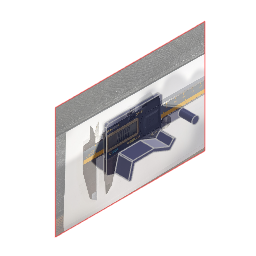
caliper stand (Autodesk Fusion 360 design; units mm, degrees)
Autodesk Fusion 360 part; units mm, degrees
sketch "Sketch1" plane through (0, 0, 0) normal (1, 0, 0) x (0, 1, 0)
  line L0 (-5.19, -7.01) -> (-3.78, -7)
  line L1 (-13, -16.1) -> (11.5, -15.8)
  line L2 (27.8164, -22.4078) -> (11.5, -15.8)
  line L3 (27.8164, -22.4078) -> (31.6352, -18.1647)
  line L4 (-13, -16.1) -> (-17.5, -34)
  line L5 (-12.7967, -17.3419) -> (-16.7713, -33.1521)
  line L6 (-11.8391, -16.5858) -> (11.2044, -16.3037)
  line L7 (27.9536, -23.0028) -> (11.592, -16.3767)
  line L8 (27.9536, -23.0028) -> (32.7851, -17.6344)
  line L9 (-10.0593, -20.8087) -> (-13.3769, -34.0054)
  line L10 (-9.1017, -20.0526) -> (10.5432, -19.812)
  line L11 (28.2641, -26.9047) -> (10.9308, -19.8851)
  line L12 (29.3828, -26.6468) -> (35.3866, -19.9758)
  arc A0 (-11.8391, -16.5858) -> (-12.7967, -17.3419) centre (-11.8268, -17.5857) ccw
  arc A1 (11.592, -16.3767) -> (11.2044, -16.3037) centre (11.2166, -17.3036) ccw
  arc A2 (28.2641, -26.9047) -> (29.3828, -26.6468) centre (28.6395, -25.9778) ccw
  arc A3 (-9.1017, -20.0526) -> (-10.0593, -20.8087) centre (-9.0895, -21.0525) ccw
  arc A4 (10.9308, -19.8851) -> (10.5432, -19.812) centre (10.5555, -20.8119) ccw
  line L13 (-16.0453, -34.3657) -> (-14.5905, -34.7314)
  line L14 (35.3123, -18.5635) -> (34.1974, -17.5601)
  arc A5 (34.1974, -17.5601) -> (32.7851, -17.6344) centre (33.5284, -18.3034) ccw
  arc A6 (35.3866, -19.9758) -> (35.3123, -18.5635) centre (34.6433, -19.3068) ccw
  arc A7 (-16.7713, -33.1521) -> (-16.0453, -34.3657) centre (-15.8015, -33.3959) ccw
  arc A8 (-14.5905, -34.7314) -> (-13.3769, -34.0054) centre (-14.3467, -33.7616) ccw
  circle A9 centre (57, -12.25) radius 4
  dimension "d4" = 1
  dimension "d5" = 1
  dimension "d34" = 8
  dimension "d41" = 12.25
  dimension "d42" = 57
  constraint parallel L4 L5
  constraint parallel L1 L6
  constraint parallel L2 L7
  constraint parallel L3 L8
  constraint tangent L6 A0
  constraint tangent L5 A0
  constraint tangent L6 A1
  constraint tangent L7 A1
  constraint equal A0 A1
  constraint parallel L4 L9
  constraint parallel L1 L10
  constraint parallel L2 L11
  constraint parallel L3 L12
  constraint tangent L12 A2
  constraint tangent L11 A2
  constraint equal A0 A2
  constraint tangent L10 A3
  constraint tangent L9 A3
  constraint equal A0 A3
  constraint tangent L10 A4
  constraint tangent L11 A4
  constraint equal A0 A4
  constraint perpendicular L9 L13
  constraint perpendicular L8 L14
  constraint tangent L8 A5
  constraint tangent L14 A5
  constraint tangent L12 A6
  constraint tangent L14 A6
  constraint equal A5 A6
  constraint tangent L13 A7
  constraint tangent L5 A7
  constraint equal A5 A7
  constraint tangent L13 A8
  constraint tangent L9 A8
  constraint equal A5 A8
  measures "d4" radius of A0
  measures "d5" radius of A5
  measures "d34" diameter of A9
  measures "d41" vertical distance of origin A9.centre
  measures "d42" horizontal distance of origin A9.centre
extrude "Extrude1" add sketch "Sketch1" along normal blind 15 makes body 1 at (5, -4.1579, -16.4918) makes body 2 at (10, 60.9801, -12.6483)
sketch "Sketch3" plane through (0, 0, 0) normal (1, 0, 0) x (0, 1, 0)
  line L0 (28.2641, -26.9047) -> (10.9308, -19.8851)
  arc A0 (28.2641, -26.9047) -> (29.3828, -26.6468) centre (28.6395, -25.9778) ccw
  line L1 (29.3828, -26.6468) -> (35.3866, -19.9758)
  line L2 (-9.1017, -20.0526) -> (10.5432, -19.812)
  line L3 (-10.0593, -20.8087) -> (-13.3769, -34.0054)
  arc A1 (-9.1017, -20.0526) -> (-10.0593, -20.8087) centre (-9.0895, -21.0525) ccw
  arc A2 (-14.5905, -34.7314) -> (-13.3769, -34.0054) centre (-14.3467, -33.7616) ccw
  line L4 (-16.0453, -34.3657) -> (-14.5905, -34.7314)
  arc A3 (-16.7713, -33.1521) -> (-16.0453, -34.3657) centre (-15.8015, -33.3959) ccw
  line L5 (-12.7967, -17.3419) -> (-16.7713, -33.1521)
  line L6 (35.3866, 7.7018) -> (35.3866, 14)
  line L7 (32.3866, 17) -> (-23, 17)
  line L8 (-26, 14) -> (-26, -29.524)
  line L9 (-23.7314, -32.4334) -> (-16.0453, -34.3657)
  arc A4 (-26, -29.524) -> (-23.7314, -32.4334) centre (-23, -29.524) ccw
  arc A5 (-23, 17) -> (-26, 14) centre (-23, 14) ccw
  arc A6 (35.3866, 14) -> (32.3866, 17) centre (32.3866, 14) ccw
  line L10 (35.3866, -19.9758) -> (29.3828, -26.6468)
  line L11 (28.2641, -26.9047) -> (10.9308, -19.8851)
  line L12 (-9.1017, -20.0526) -> (10.5432, -19.812)
  line L13 (-10.0593, -20.8087) -> (-13.3769, -34.0054)
  line L14 (-14.5905, -34.7314) -> (-16.0453, -34.3657)
  arc A7 (28.2641, -26.9047) -> (29.3828, -26.6468) centre (28.6395, -25.9778) ccw
  arc A8 (10.9308, -19.8851) -> (10.5432, -19.812) centre (10.5555, -20.8119) ccw
  arc A9 (10.9308, -19.8851) -> (10.5432, -19.812) centre (10.5555, -20.8119) ccw
  arc A10 (-9.1017, -20.0526) -> (-10.0593, -20.8087) centre (-9.0895, -21.0525) ccw
  arc A11 (-14.5905, -34.7314) -> (-13.3769, -34.0054) centre (-14.3467, -33.7616) ccw
  line L15 (-10, 17) -> (-10, 14)
  line L16 (-10, 14) -> (-26, 14)
  circle A12 centre (57, -12.25) radius 4
  line L17 (57, -16.25) -> (36.3866, -16.25)
  line L18 (59.3943, -9.0457) -> (37.8866, 3.3717)
  arc A13 (35.3866, 7.7018) -> (37.8866, 3.3717) centre (40.3866, 7.7018) ccw
  line L19 (35.3866, -19.9758) -> (35.3866, -17.25)
  arc A14 (36.3866, -16.25) -> (35.3866, -17.25) centre (36.3866, -17.25) ccw
  arc A15 (57, -16.25) -> (59.3943, -9.0457) centre (57, -12.25) ccw
  point P0 (-16.0453, -34.3657)
  dimension "d8" = 3
  dimension "d35" = 30
  dimension "d36" = 5
  dimension "d37" = 1
  constraint vertical L6
  constraint perpendicular L6 L7
  constraint perpendicular L7 L8
  constraint coincident P0 L4.start
  constraint collinear L4 L9
  constraint tangent L9 A4
  constraint tangent L8 A4
  constraint tangent L8 A5
  constraint tangent L7 A5
  constraint equal A4 A5
  constraint tangent L7 A6
  constraint tangent L6 A6
  constraint equal A4 A6
  constraint coincident L1.end L10.start
  constraint coincident A0.end L1.start
  constraint coincident L0.start A0.start
  constraint coincident L0.end L11.end
  constraint coincident L2.start A1.start
  constraint coincident L2.end L12.end
  constraint coincident L3.start A1.end
  constraint coincident L3.end A2.end
  constraint coincident A2.start L4.end
  constraint coincident A0.centre A7.centre
  constraint coincident A2.centre A11.centre
  constraint coincident L7 L15.start
  constraint perpendicular L7 L15
  constraint coincident A12 L17.start
  constraint tangent A12 L17
  constraint horizontal L17
  constraint coincident A12 L18.start
  constraint tangent L18 A13
  constraint tangent L6 A13
  constraint perpendicular L17 L19
  constraint tangent L19 A14
  constraint tangent L17 A14
  constraint coincident A12.centre A15.centre
  measures "d8" radius of A4
  measures "d35" angle of L17 L18
  measures "d36" radius of A13
  measures "d37" radius of A14
extrude "Extrude2" add sketch "Sketch3" against normal blind 3 contours L0 A0 L1 L2 L3 A1 A2 L4 L6 L7 L8 L9 A4 A6 L10 L11 L12 L13 L14 A7 A8 A9 A10 A11 L15 L16 A12 L17 L18 A13 L19 A14 | A12 L18 A15 | L7 A5 L15 L16 bodies 1 2
ref_plane "WorkPlane1" through (0, 12.125, 0) normal (0.34202, 0, 0.939693) x (0, 1, 0)
sketch "Sketch4" plane through (0, 12.125, 0) normal (0.34202, 0, 0.939693) x (0, 1, 0)
  ellipse E0 centre (-35.125, 4.7883) end of major axis (-38.125, 4.7883) minor radius 1.0261 (-35.125, 5.8143) -> (-38.125, 4.7883) ccw
  line L0 (-35.125, 5.8143) -> (-35.125, 8.6334)
  ellipse E1 centre (-35.125, 7.6074) end of major axis (-38.125, 7.6074) minor radius 1.0261 (-35.125, 8.6334) -> (-38.125, 7.6074) ccw
  line L1 (-38.125, 7.6074) -> (-38.125, 4.7883)
  line L2 (-35.125, 5.8143) -> (20.2616, 5.8143)
  line L3 (20.2616, 5.8143) -> (20.2616, 8.6334)
  line L4 (20.2616, 8.6334) -> (-35.125, 8.6334)
  ellipse E2 centre (20.2616, 4.7883) end of major axis (23.2616, 4.7883) minor radius 1.0261 (23.2616, 4.7883) -> (20.2616, 5.8143) ccw
  line L5 (23.2616, 4.7883) -> (23.2616, 7.6074)
  ellipse E3 centre (20.2616, 7.6074) end of major axis (23.2616, 7.6074) minor radius 1.0261 (23.2616, 7.6074) -> (20.2616, 8.6334) ccw
  line L6 (20.2616, 8.6334) -> (20.2616, 5.8143)
  ellipse E4 centre (22.5183, -6.6033) end of major axis (21.5183, -6.6033) minor radius 0.342 (23.2616, -6.3745) -> (23.1873, -6.3491) ccw
  line L7 (23.2616, 2.6342) -> (23.2616, 4.7883)
  ellipse E5 centre (20.2616, 4.7883) end of major axis (23.2616, 4.7883) minor radius 1.0261 (23.2616, 4.7883) -> (20.2616, 5.8143) ccw
  line L8 (20.2616, 5.8143) -> (-35.125, 5.8143)
  line L9 (-38.125, 4.7883) -> (-38.125, -10.0978)
  ellipse E6 centre (-35.125, -10.0978) end of major axis (-38.125, -10.0978) minor radius 1.0261 (-38.125, -10.0978) -> (-35.8564, -11.0929) ccw
  line L10 (-35.8564, -11.0929) -> (-28.1703, -11.7538)
  ellipse E7 centre (-27.9265, -11.4221) end of major axis (-28.9265, -11.4221) minor radius 0.342 (-28.8963, -11.3387) -> (-28.1703, -11.7538) ccw
  line L11 (-28.8963, -11.3387) -> (-24.9217, -5.9313)
  ellipse E8 centre (-23.9518, -6.0147) end of major axis (-24.9518, -6.0147) minor radius 0.342 (-23.9641, -5.6727) -> (-24.9217, -5.9313) ccw
  line L12 (-23.9641, -5.6727) -> (-0.9206, -5.5762)
  ellipse E9 centre (-0.9084, -5.9182) end of major axis (-1.9084, -5.9182) minor radius 0.342 (-0.533, -5.6012) -> (-0.9206, -5.5762) ccw
  line L13 (-0.533, -5.6012) -> (15.8286, -7.8674)
  line L14 (15.8286, -7.8674) -> (20.6601, -6.0313)
  ellipse E10 centre (21.4034, -6.2601) end of major axis (20.4034, -6.2601) minor radius 0.342 (22.0724, -6.0059) -> (20.6601, -6.0313) ccw
  line L15 (22.0724, -6.0059) -> (23.1873, -6.3491)
  line L16 (-35.125, 8.6334) -> (20.2616, 8.6334)
  line L17 (20.2616, 8.6334) -> (20.2616, 0.6334)
  line L18 (20.2616, 0.6334) -> (-35.125, 0.6334)
  line L19 (-35.125, 0.6334) -> (-35.125, 8.6334)
  line L20 (23.2616, -6.3745) -> (23.2616, -5.8998)
  ellipse E11 centre (24.2616, -5.8998) end of major axis (23.2616, -5.8998) minor radius 0.342 (24.2616, -5.5578) -> (23.2616, -5.8998) ccw
  line L21 (24.2616, -5.5578) -> (44.875, -5.5578)
  line L22 (46.4528, -2.9326) -> (25.7616, 1.1532)
  ellipse E12 centre (28.2616, 2.6342) end of major axis (23.2616, 2.6342) minor radius 1.7101 (23.2616, 2.6342) -> (25.7616, 1.1532) ccw
  line L23 (-35.125, 8.6334) -> (-35.125, 5.8143)
  ellipse E13 centre (-35.125, 4.7883) end of major axis (-38.125, 4.7883) minor radius 1.0261 (-35.125, 5.8143) -> (-38.125, 4.7883) ccw
  ellipse E14 centre (44.875, -4.1897) end of major axis (40.875, -4.1897) minor radius 1.3681 (46.4528, -2.9326) -> (44.875, -5.5578) ccw
  dimension "d12" = 8
  constraint perpendicular L16 L17
  constraint parallel L16 L18
  constraint parallel L17 L19
  constraint coincident L3.end L4.start
  constraint perpendicular L3 L16
  constraint coincident L0.end L4.end
  measures "d12" distance of L0.end L18.end
ref_plane "WorkPlane2" through (-11.6287, 12.125, -31.9495) normal (0.34202, 0, 0.939693) x (0, 1, 0)
sketch "Sketch5" plane through (-11.6287, 12.125, -31.9495) normal (0.34202, 0, 0.939693) x (0, 1, 0)
  ellipse E0 centre (-35.125, 4.7883) end of major axis (-38.125, 4.7883) minor radius 1.0261 (-35.125, 5.8143) -> (-38.125, 4.7883) ccw
  line L0 (-35.125, 5.8143) -> (-35.125, 8.6334)
  ellipse E1 centre (-35.125, 7.6074) end of major axis (-38.125, 7.6074) minor radius 1.0261 (-35.125, 8.6334) -> (-38.125, 7.6074) ccw
  line L1 (-38.125, 7.6074) -> (-38.125, 4.7883)
  line L2 (-35.125, 5.8143) -> (20.2616, 5.8143)
  line L3 (20.2616, 5.8143) -> (20.2616, 8.6334)
  line L4 (20.2616, 8.6334) -> (-35.125, 8.6334)
  ellipse E2 centre (20.2616, 4.7883) end of major axis (23.2616, 4.7883) minor radius 1.0261 (23.2616, 4.7883) -> (20.2616, 5.8143) ccw
  line L5 (23.2616, 4.7883) -> (23.2616, 7.6074)
  ellipse E3 centre (20.2616, 7.6074) end of major axis (23.2616, 7.6074) minor radius 1.0261 (23.2616, 7.6074) -> (20.2616, 8.6334) ccw
  line L6 (20.2616, 8.6334) -> (20.2616, 5.8143)
  ellipse E4 centre (22.5183, -6.6033) end of major axis (21.5183, -6.6033) minor radius 0.342 (23.2616, -6.3745) -> (23.1873, -6.3491) ccw
  line L7 (23.2616, 2.6342) -> (23.2616, 4.7883)
  ellipse E5 centre (20.2616, 4.7883) end of major axis (23.2616, 4.7883) minor radius 1.0261 (23.2616, 4.7883) -> (20.2616, 5.8143) ccw
  line L8 (20.2616, 5.8143) -> (-35.125, 5.8143)
  line L9 (-38.125, 4.7883) -> (-38.125, -10.0978)
  ellipse E6 centre (-35.125, -10.0978) end of major axis (-38.125, -10.0978) minor radius 1.0261 (-38.125, -10.0978) -> (-35.8564, -11.0929) ccw
  line L10 (-35.8564, -11.0929) -> (-28.1703, -11.7538)
  ellipse E7 centre (-27.9265, -11.4221) end of major axis (-28.9265, -11.4221) minor radius 0.342 (-28.8963, -11.3387) -> (-28.1703, -11.7538) ccw
  line L11 (-28.8963, -11.3387) -> (-24.9217, -5.9313)
  ellipse E8 centre (-23.9518, -6.0147) end of major axis (-24.9518, -6.0147) minor radius 0.342 (-23.9641, -5.6727) -> (-24.9217, -5.9313) ccw
  line L12 (-23.9641, -5.6727) -> (-0.9206, -5.5762)
  ellipse E9 centre (-0.9084, -5.9182) end of major axis (-1.9084, -5.9182) minor radius 0.342 (-0.533, -5.6012) -> (-0.9206, -5.5762) ccw
  line L13 (-0.533, -5.6012) -> (15.8286, -7.8674)
  line L14 (15.8286, -7.8674) -> (20.6601, -6.0313)
  ellipse E10 centre (21.4034, -6.2601) end of major axis (20.4034, -6.2601) minor radius 0.342 (22.0724, -6.0059) -> (20.6601, -6.0313) ccw
  line L15 (22.0724, -6.0059) -> (23.1873, -6.3491)
  line L16 (-35.125, 8.6334) -> (20.2616, 8.6334)
  line L17 (20.2616, 8.6334) -> (20.2616, 0.6334)
  line L18 (20.2616, 0.6334) -> (-35.125, 0.6334)
  line L19 (-35.125, 0.6334) -> (-35.125, 8.6334)
  line L20 (23.2616, -6.3745) -> (23.2616, -5.8998)
  ellipse E11 centre (24.2616, -5.8998) end of major axis (23.2616, -5.8998) minor radius 0.342 (24.2616, -5.5578) -> (23.2616, -5.8998) ccw
  line L21 (24.2616, -5.5578) -> (44.875, -5.5578)
  line L22 (46.4528, -2.9326) -> (25.7616, 1.1532)
  ellipse E12 centre (28.2616, 2.6342) end of major axis (23.2616, 2.6342) minor radius 1.7101 (23.2616, 2.6342) -> (25.7616, 1.1532) ccw
  line L23 (-35.125, 8.6334) -> (-35.125, 5.8143)
  ellipse E13 centre (-35.125, 4.7883) end of major axis (-38.125, 4.7883) minor radius 1.0261 (-35.125, 5.8143) -> (-38.125, 4.7883) ccw
  ellipse E14 centre (44.875, -4.1897) end of major axis (40.875, -4.1897) minor radius 1.3681 (46.4528, -2.9326) -> (44.875, -5.5578) ccw
  dimension "d14" = 8
  constraint perpendicular L16 L17
  constraint parallel L16 L18
  constraint parallel L17 L19
  constraint coincident L3.end L4.start
  constraint tangent E1 L16
  constraint coincident L0.end L4.end
  measures "d14" distance of L0.end L18.end
extrude "Extrude3" add sketch "Sketch5" along normal up to surface contours L0 L2 L3 L4 L6 L8 L16 L17 L19 L23 | L2 L8 L17 L18 L19 end surface through (-3, 0, 0) normal (-1, 0, 0) offset 0 bodies 1
sketch "Sketch6" plane through (0, 32.3866, 0) normal (0, 1, 0) x (-1, 0, 0)
  line L0 (3, 17) -> (3, -6.3904)
  line L1 (3, -6.3904) -> (12.2239, -31.7329)
  line L2 (12.2239, -31.7329) -> (19.7414, -28.9967)
  line L3 (19.7414, -28.9967) -> (3, 17)
  line L4 (3, 7.7018) -> (3, 14)
extrude "Extrude4" add sketch "Sketch6" against normal up to surface (55.3866 mm away) bodies 1
sketch "Sketch8" plane through (-3, 0, 0) normal (-1, 0, 0) x (0, -1, 0)
  line L0 (-32.3866, -6.3904) -> (-32.3866, 17)
  arc A0 (-32.3866, 17) -> (-35.3866, 14) centre (-32.3866, 14) ccw
  line L1 (-35.3866, 14) -> (-35.3866, 7.7018)
  line L2 (-35.3866, -19.9758) -> (-29.3828, -26.6468)
  arc A1 (-29.3828, -26.6468) -> (-28.2641, -26.9047) centre (-28.6395, -25.9778) ccw
  line L3 (-28.2641, -26.9047) -> (-10.9308, -19.8851)
  line L4 (23, -6.3904) -> (23, -31.7329)
  line L5 (23, -31.7329) -> (-32.3866, -31.7329)
  line L6 (-32.3866, -31.7329) -> (-32.3866, -6.3904)
  line L7 (10.0593, -20.8087) -> (13.3769, -34.0054)
  arc A2 (13.3769, -34.0054) -> (14.5905, -34.7314) centre (14.3467, -33.7616) ccw
  line L8 (14.5905, -34.7314) -> (23.7314, -32.4334)
  arc A3 (23.7314, -32.4334) -> (26, -29.524) centre (23, -29.524) ccw
  line L9 (26, -29.524) -> (26, 14)
  line L10 (23, 17) -> (23, -6.3904)
  line L11 (-10.5432, -19.812) -> (9.1017, -20.0526)
  arc A4 (10.0593, -20.8087) -> (9.1017, -20.0526) centre (9.0895, -21.0525) ccw
  arc A5 (-37.8866, 3.3717) -> (-35.3866, 7.7018) centre (-40.3866, 7.7018) ccw
  line L12 (-37.8866, 3.3717) -> (-59.3943, -9.0457)
  arc A6 (-59.3943, -9.0457) -> (-57, -16.25) centre (-57, -12.25) ccw
  line L13 (-57, -16.25) -> (-36.3866, -16.25)
  arc A7 (-35.3866, -17.25) -> (-36.3866, -16.25) centre (-36.3866, -17.25) ccw
  line L14 (-35.3866, -17.25) -> (-35.3866, -19.9758)
  arc A8 (26, 14) -> (23, 17) centre (23, 14) ccw
  arc A9 (-10.5432, -19.812) -> (-10.9308, -19.8851) centre (-10.5555, -20.8119) ccw
  line L15 (-10.5432, -19.812) -> (9.1017, -20.0526)
  arc A10 (10.0593, -20.8087) -> (9.1017, -20.0526) centre (9.0895, -21.0525) ccw
  line L16 (10.0593, -20.8087) -> (13.3769, -34.0054)
  arc A11 (13.3769, -34.0054) -> (14.5905, -34.7314) centre (14.3467, -33.7616) ccw
  line L17 (14.5905, -34.7314) -> (23.7314, -32.4334)
  arc A12 (23.7314, -32.4334) -> (26, -29.524) centre (23, -29.524) ccw
  line L18 (26, -29.524) -> (26, 14)
  arc A13 (26, 14) -> (23, 17) centre (23, 14) ccw
  line L19 (23, 17) -> (23, -6.3904)
  line L20 (23, -6.3904) -> (-32.3866, -6.3904)
  line L21 (-32.3866, -6.3904) -> (23, -6.3904)
  line L22 (-32.3866, -6.3904) -> (-32.3866, 17)
  arc A14 (-32.3866, 17) -> (-35.3866, 14) centre (-32.3866, 14) ccw
  line L23 (-35.3866, 14) -> (-35.3866, 7.7018)
  arc A15 (-37.8866, 3.3717) -> (-35.3866, 7.7018) centre (-40.3866, 7.7018) ccw
  line L24 (-37.8866, 3.3717) -> (-59.3943, -9.0457)
  arc A16 (-59.3943, -9.0457) -> (-57, -16.25) centre (-57, -12.25) ccw
  line L25 (-57, -16.25) -> (-36.3866, -16.25)
  arc A17 (-35.3866, -17.25) -> (-36.3866, -16.25) centre (-36.3866, -17.25) ccw
  line L26 (-35.3866, -17.25) -> (-35.3866, -19.9758)
  line L27 (-35.3866, -19.9758) -> (-29.3828, -26.6468)
  arc A18 (-29.3828, -26.6468) -> (-28.2641, -26.9047) centre (-28.6395, -25.9778) ccw
  line L28 (-28.2641, -26.9047) -> (-10.9308, -19.8851)
  arc A19 (-10.5432, -19.812) -> (-10.9308, -19.8851) centre (-10.5555, -20.8119) ccw
  line L29 (23, -6.3904) -> (-32.3866, -6.3904)
extrude "Extrude5" add sketch "Sketch8" along normal up to surface contours L2 A1 L3 L4 L5 L6 L7 L11 A4 A9 L15 A10 L16 L20 L21 L27 A18 L28 A19 L29 end surface through (-12.2239, 32.3866, -31.7329) normal (0.939693, 0, -0.34202) offset 0 bodies 1
sketch "Sketch7" plane through (-0.5952, 0, 0.2166) normal (0.939693, 0, -0.34202) x (0, 1, 0)
  line L0 (-12.8056, -34) -> (32.3866, -34)
  line L1 (32.3866, -34) -> (32.3866, -25.0356)
  line L2 (33.0271, -28) -> (-22.3596, -28) construction
  line L3 (32.3866, -25.0356) -> (29.3828, -28.5874)
  ellipse E0 centre (28.6395, -27.8755) end of major axis (28.6395, -28.9397) minor radius 1 (28.2641, -28.8619) -> (29.3828, -28.5874) ccw
  line L4 (28.2641, -28.8619) -> (10.9308, -21.3918)
  ellipse E1 centre (10.5555, -22.3782) end of major axis (10.5555, -21.314) minor radius 1 (10.9308, -21.3918) -> (10.5432, -21.3141) ccw
  line L5 (10.5432, -21.3141) -> (-9.1017, -21.57)
  ellipse E2 centre (-9.0895, -22.6341) end of major axis (-9.0895, -21.57) minor radius 1 (-9.1017, -21.57) -> (-10.0593, -22.3747) ccw
  line L6 (-10.0593, -22.3747) -> (-12.8056, -34)
  point P0 (-8, -28)
  point P1 (17.3866, -28)
  dimension "d20" = 15
  dimension "d38" = 6
  constraint coincident L2 P0
  constraint coincident L2 P1
  constraint horizontal L2
  measures "d20" distance of L1 P1
  measures "d38" distance of L0 L2
hole "Hole1" at (-10.1718, -8, -26.0948) at (-10.1718, 17.3866, -26.0948) direction (-0.939693, 0, 0.34202) diameter 5.5 end through all countersink diameter 10.4 countersink angle 90 bodies 1
sketch "Sketch10" plane through (-0.5952, 0, 0.2166) normal (0.939693, 0, -0.34202) x (0, 1, 0)
  arc A0 (-12.1335, -31.155) -> (-10.2847, -23.3288) centre (-8, -28) ccw
  line L0 (-12.1335, -31.155) -> (-12.8056, -34)
  line L1 (-12.8056, -34) -> (32.3866, -34)
  line L2 (32.3866, -34) -> (32.3866, -25.0356)
  line L3 (32.3866, -25.0356) -> (29.3828, -28.5874)
  ellipse E0 centre (28.6395, -27.8755) end of major axis (28.6395, -28.9397) minor radius 1 (28.2641, -28.8619) -> (29.3828, -28.5874) ccw
  line L4 (28.2641, -28.8619) -> (22.2976, -26.2905)
  arc A1 (15.2568, -23.2562) -> (22.2976, -26.2905) centre (17.3866, -28) ccw
  line L5 (15.2568, -23.2562) -> (10.9308, -21.3918)
  ellipse E1 centre (10.5555, -22.3782) end of major axis (10.5555, -21.314) minor radius 1 (10.9308, -21.3918) -> (10.5432, -21.3141) ccw
  line L6 (10.5432, -21.3141) -> (-9.1017, -21.57)
  ellipse E2 centre (-9.0895, -22.6341) end of major axis (-9.0895, -21.57) minor radius 1 (-9.1017, -21.57) -> (-10.0593, -22.3747) ccw
  line L7 (-10.0593, -22.3747) -> (-10.2847, -23.3288)
  arc A2 (15.2568, -23.2562) -> (22.2976, -26.2905) centre (17.3866, -28) ccw
  arc A3 (-12.1335, -31.155) -> (-10.2847, -23.3288) centre (-8, -28) ccw
  circle A4 centre (-8, -28) radius 5.2
  circle A5 centre (17.3866, -28) radius 5.2
  constraint concentric A3 A4
  constraint concentric A2 A5
  constraint equal A0 A4
  constraint equal A1 A5
extrude "Extrude9" cut sketch "Sketch10" along normal blind 29 contours A0 A3 A4 | A1 A2 A5 bodies 1
extrude "Extrude8" [suppressed]
